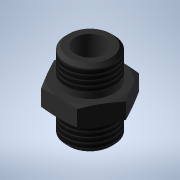
# Autodesk Inventor part: 8030272 NPFC-D-2G14-M
Saved by Autodesk Inventor 2021 (Build 250183000, 183)
## iProperties
Created: 2026-09-15
Part Number: 8030272 NPFC-D-2G14-M
Material: Generic
Catalog Web Link: www.3dfindit.com
Description: NPFC-D-Double nipple
Vendor: FESTO
Document SubType Name: Modeling
Designer: psAdmin
Manufacturer: FESTO
Mass: 17.2 g
Surface Area: 18.2766 cm^2
Volume: 2.33723 cm^3
Density: 1 g/cm^3
Appearance: PSOLRGB-176-176-176
Category: PARTsolutions
Company: FESTO
Title: 8030272 NPFC-D-2G14-M
Author: Cadenas PARTsolutions
Comments: Double nipple
PSOL_IDENT_0: {$CADENAS_DATA/23d-libs/festo/parts/n/npfc/npfc_d.prj},183 {VTYP=3D},{NB=8030272 NPFC-D-2G14-M},{LIN
PSOL_IDENT_1: A=8030272 NPFC-D-2G14-M},{NN=NPFC-D},{DATE=05.05.2026 12:08:01},{GEOMDATE=31.03.2025 12:43:22},{VERS
PSOL_IDENT_2: ION=},{LINEID=900},{WBVAR=},{WBNUMERIC=}  {NB=8030272 NPFC-D-2G14-M},{LINA=8030272 NPFC-D-2G14-M},{K
PSOL_IDENT_3: T=DUMMY},{TNR=8030272},{TYP=NPFC-D-2G14-M},{VERS=15},{D=8.0},{T1=G1/4},{T1C=13.157},{T2=G1/4},{T2C=1
PSOL_IDENT_4: 3.157},{A1=8.0},{A2=8.0},{B=21.00},{SW=17},{CNSMASSEXACT=0.01720},{VERS2=3},{GTIN=4052568063740},{RE
PSOL_IDENT_5: ACH=Ja},{REACHSVHC=Ja},{REACHHAZSUBS=7439-92-1},{REACHSCIP=6d587698-b8b9-4b84-bce2-6775519e5c5d},{RE
PSOL_IDENT_6: ACHVALDATE=05.03.2025}
NB: 8030272 NPFC-D-2G14-M
NN: NPFC-D
NT: Double nipple
NBSYN: $TNR. $TYP.
LINA: 8030272 NPFC-D-2G14-M
CATALOG: Festo
TNR: 8030272
TYP: NPFC-D-2G14-M
D: 8
T1: G1/4
T2: G1/4
A1: 8
A2: 8
B: 21
SW: 17
CNSMASSEXACT: 0.0172
GTIN: 4052568063740
REACH: Yes
REACHSVHC: Yes
REACHHAZSUBS: 7439-92-1
REACHVALDATE: 05.03.2025
SUPPLIER: FESTO
ARTICLENO: 8030272 NPFC-D-2G14-M
BOMINFO: 8030272 NPFC-D-2G14-M
CREATOR: CADENAS GmbH
Autodesk Inventor part; units mm, degrees
sketch "Sketch_6" plane through (0, 0, 0) normal (0, 0, 1) x (1, 0, 0)
  line L0 (0, 0) -> (0, 13)
  line L1 (0, 13) -> (8.5, 13)
  line L2 (8.5, 13) -> (10.2, 12.5445)
  line L3 (10.2, 12.5445) -> (10.2, 8.4555)
  line L4 (10.2, 8.4555) -> (8.5, 8)
  line L5 (8.5, 8) -> (6.5785, 8)
  line L6 (6.5785, 8) -> (6.5785, 0.856)
  line L7 (6.5785, 0.856) -> (5.7225, 0)
  line L8 (5.7225, 0) -> (0, 0)
  line L9 (0, 0) -> (0, 13)
  constraints: 20 end point
revolve "Revolution1" add sketch "Sketch_6" angle 360 about axis through (0, 0, 0) along (0, -1, 0)
thread "Thread1" size "G13.157x1.337" designation "G 1/4" class "A" standard "ISO Pipe Threads" length 5.544
sketch "Sketch_7" plane through (0, 0, 0) normal (0, 0, 1) x (1, 0, 0)
  line L0 (0, 13) -> (0, 21)
  line L1 (0, 21) -> (5.7225, 21)
  line L2 (5.7225, 21) -> (6.5785, 20.144)
  line L3 (6.5785, 20.144) -> (6.5785, 13)
  line L4 (6.5785, 13) -> (0, 13)
  line L5 (0, 13) -> (0, 21)
  constraints: 12 end point
revolve "Revolution2" add sketch "Sketch_7" angle 360 about axis through (0, 13, 0) along (0, -1, 0)
thread "Thread2" size "G13.157x1.337" designation "G 1/4" class "A" standard "ISO Pipe Threads" length 5.544
sketch "Sketch_10" plane through (0, 10.5, 0) normal (0, 1, 0) x (1, 0, 0)
  line L0 (-17, -17) -> (17, -17)
  line L1 (17, -17) -> (17, 17)
  line L2 (17, 17) -> (-17, 17)
  line L3 (-17, 17) -> (-17, -17)
  line L4 (-9.815, 0) -> (-4.9075, -8.5)
  line L5 (-4.9075, -8.5) -> (4.9075, -8.5)
  line L6 (4.9075, -8.5) -> (9.815, 0)
  line L7 (9.815, 0) -> (4.9075, 8.5)
  line L8 (4.9075, 8.5) -> (-4.9075, 8.5)
  line L9 (-4.9075, 8.5) -> (-9.815, 0)
  constraints: 20 end point
extrude "Extrusion1" cut sketch "Sketch_10" along normal mid plane 12.6
sketch "Sketch4" plane through (0, 0, 0) normal (0, -1, 0) x (1, 0, 0)
  point P0 (0, 0)
hole "Hole1" at (0, 0, 0) direction (0, 1, 0) diameter 8 depth 21
ref_plane "IP1_XY" through (0, 0, 0) normal (0, 1, 0) x (1, 0, 0)
ref_plane "IP1_YZ" through (0, 0, 0) normal (1, 0, 0) x (0, 0, -1)
ref_plane "IP1_ZX" through (0, 0, 0) normal (0, 0, -1) x (0, 1, 0)
ref_plane "IP2_XY" through (0, 21, 0) normal (0, -1, 0) x (1, 0, 0)
ref_plane "IP2_YZ" through (0, 21, 0) normal (1, 0, 0) x (0, 0, 1)
ref_plane "IP2_ZX" through (0, 21, 0) normal (0, 0, 1) x (0, -1, 0)
ref_plane "RING1_XY" through (0, 8, 0) normal (0, 1, 0) x (1, 0, 0)
ref_plane "RING1_YZ" through (0, 8, 0) normal (1, 0, 0) x (0, 0, -1)
ref_plane "RING1_ZX" through (0, 8, 0) normal (0, 0, -1) x (0, 1, 0)
ref_plane "RING2_XY" through (0, 13, 0) normal (0, -1, 0) x (1, 0, 0)
ref_plane "RING2_YZ" through (0, 13, 0) normal (1, 0, 0) x (0, 0, 1)
ref_plane "RING2_ZX" through (0, 13, 0) normal (0, 0, 1) x (0, -1, 0)
body "Solid1"
